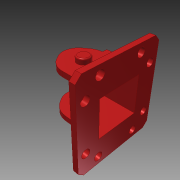
# Autodesk Inventor part: z_axis_cable_mount_b
Saved by Autodesk Inventor 2014 (Build 180170000, 170)
## iProperties
Created: 2013-12-04
Part Number: z_axis_cable_mount_b
Material: ABS Plastic
Document SubType Name: Modeling
Designer: buben
Density: 1.06 g/cm^3
Appearance: Light Red
Author: buben
Autodesk Inventor part; units mm, degrees
ref_plane "YZ Plane" through (0, 0, 0) normal (1, 0, 0) x (0, 1, 0)
sketch "Sketch1" plane through (0, 0, 0) normal (0, 0, 1) x (1, 0, 0)
  circle A0 centre (0, 0) radius 2.5
  circle A1 centre (20, 0) radius 2.5
  line L0 (7, 10) -> (20, 10)
  line L1 (7, -10) -> (20, -10)
  arc A2 (20, -10) -> (20, 10) centre (20, 0) ccw
  line L2 (7, 10) -> (7, 8)
  line L3 (7, -10) -> (7, -8)
  line L4 (7, 8) -> (0, 8)
  line L5 (7, -8) -> (0, -8)
  arc A3 (0, 8) -> (0, -8) centre (0, 0) ccw
  dimension "d0" = 5
  dimension "d1" = 20
  dimension "d2" = 10
  dimension "d3" = 2
  dimension "d4" = 13
  constraints: 12 end point, 4 centre point, 4 point on circle, 4 tangent, 3 parallel, 2 collinear, 2 concentric, 1 coincident, 1 equal radius, 1 horizontal, 1 horizontal alignment, 1 perpendicular
  measures "d0" diameter of A0
  measures "d1" distance of A1.centre point (0, 0)
  measures "d2" radius of A2
  measures "d3" distance of L0.start L2.end
  measures "d4" distance from line of L2 A1.centre
extrude "Extrusion1" add sketch "Sketch1" along normal blind 4
sketch "Sketch2" plane through (0, 0, 4) normal (0, 0, 1) x (1, 0, 0)
  circle A0 centre (0, 0) radius 2.5 projected
  line L0 (7, 8) -> (0, 8) projected
  arc A1 (0, 8) -> (0, -8) centre (0, 0) ccw projected
  line L1 (0, -8) -> (7, -8) projected
  line L2 (7, -10) -> (20, -10) projected
  line L3 (7, 8) -> (7, -8)
  line L4 (7, -8) -> (0, -8)
  line L5 (7, 8) -> (0, 8)
  arc A2 (0, 8) -> (0, -8) centre (0, 0) ccw
  constraints: 6 end point, 4 tangent, 2 collinear, 2 point on circle, 1 centre point, 1 perpendicular
extrude "Extrusion2" cut sketch "Sketch2" against normal blind 2
sketch "Sketch3" plane through (0, 0, 0) normal (0, 0, -1) x (-1, 0, 0)
  circle A0 centre (-20, 0) radius 2.5 projected
  circle A1 centre (0, 0) radius 2.5 projected
  line L0 (-7, 10) -> (-20, 10) projected
  arc A2 (-20, 10) -> (-20, -10) centre (-20, 0) ccw projected
  line L1 (-20, -10) -> (-7, -10) projected
  line L2 (-7, 8) -> (-7, 10) projected
  line L3 (-19, 10) -> (-19, 8)
  line L4 (-19, 8) -> (-11, 8)
  line L5 (-11, 8) -> (-11, -8)
  line L6 (-11, -8) -> (-19, -8)
  line L7 (-19, -8) -> (-19, -10)
  point P0 (-7, -8)
  dimension "d9" = 1
  dimension "d10" = 11
  constraints: 10 end point, 3 parallel, 2 horizontal alignment, 2 perpendicular, 2 point on line, 1 collinear
  measures "d9" distance from line of L3 A0.centre
  measures "d10" distance from line of A1.centre L5
extrude "Extrusion3" cut sketch "Sketch3" against normal blind 2 contours L3 L4 L5 L6 L7 L1 A2 L0
sketch "Sketch4" plane through (0, 0, 4) normal (0, 0, 1) x (1, 0, 0)
  line L0 (7, 10) -> (7, -10)
  circle A0 centre (0, 0) radius 2.5
  arc A1 (7, -8.485281) -> (7, 8.485281) centre (0, 0) ccw
  dimension "d15" = 11
  constraints: 2 point on circle, 2 point on line, 1 centre point, 1 coincident
  measures "d15" radius of A1
extrude "Extrusion4" cut sketch "Sketch4" against normal blind 2 contours A1 L0
sketch "Sketch5" plane through (0, 0, 0) normal (0, 0, -1) x (-1, 0, 0)
  line L0 (0, 8) -> (-7, 8) projected
  line L1 (-7, 10) -> (0, 10)
  line L2 (0, 10) -> (0, 8)
  line L3 (0, 8) -> (-7, 8)
  line L4 (-7, 8) -> (-7, 10)
  arc A0 (0, -8) -> (0, 8) centre (0, 0) ccw projected
  constraints: 8 end point, 2 parallel, 1 horizontal, 1 perpendicular, 1 point on line, 1 vertical alignment
extrude "Extrusion5" add sketch "Sketch5" against normal blind 2
sketch "Sketch6" plane through (0, 0, 0) normal (0, 0, -1) x (-1, 0, 0)
  line L0 (0, 10) -> (-19, 10) projected
  line L1 (-19, 8) -> (-20, 8)
  line L2 (-20, 8) -> (-20, 10)
  line L3 (-20, 10) -> (-19, 10)
  line L4 (-19, 10) -> (-19, 8)
  circle A0 centre (-20, 0) radius 2.5 projected
  constraints: 8 end point, 2 parallel, 1 collinear, 1 horizontal, 1 perpendicular, 1 vertical alignment
extrude "Extrusion6" add sketch "Sketch6" against normal blind 2 contours L1 L2 L3 L4
sketch "Sketch7" plane through (0, 0, 0) normal (0, 0, -1) x (-1, 0, 0)
  line L0 (-19, -8) -> (-19, -10)
  line L1 (-11, -8) -> (-19, -8)
  line L2 (-17.400642, -8) -> (-19, -9.162001)
  line L3 (-17.400642, -8) -> (-26.805206, 4.944272) construction
  line L4 (-26.805206, 4.944272) -> (-28.404564, 3.782271) construction
  line L5 (-28.404564, 3.782271) -> (-19, -9.162001) construction
  circle A0 centre (-20, 0) radius 2.5
  line L6 (-17.400642, -8) -> (-19, -8)
  line L7 (-19, -8) -> (-19, -9.162001)
  dimension "d21" = 16
  dimension "d22" = 8
  dimension "d23" = 36
  constraints: 12 end point, 3 perpendicular, 2 point on line, 1 collinear, 1 parallel
  measures "d21" distance of L2.start L3.end
  measures "d22" distance from line of A0.centre L4
  measures "d23" angle of L2 L1
extrude "Extrusion7" cut sketch "Sketch7" against normal blind 2 contours L1 L2 L0
sketch "Sketch9" plane through (0, 0, 2) normal (0, 0, 1) x (1, 0, 0)
  circle A0 centre (0, 0) radius 2.5
  arc A1 (11, 0) -> (7, 8.485281) centre (0, 0) ccw
  circle A2 centre (0, 0) radius 2.5
  constraints: 1 centre point, 1 coincident, 1 concentric
extrude "Extrusion8" add sketch "Sketch9" along normal mid plane 4
fillet "Fillet1" radius 0.5 1 edges at (-2.5, 0, 4)
sketch "Sketch10" plane through (0, 0, 0) normal (0, 0, -1) x (-1, 0, 0)
  arc A0 (0, -8) -> (0, 8) centre (0, 0) ccw
  line L0 (0, 10) -> (-20, 10)
  line L1 (4.702282, 6.472136) -> (11.174418, 1.769854)
  line L2 (11.174418, 1.769854) -> (6.472136, -4.702282)
  dimension "d30" = 144
  constraints: 4 end point, 2 point on circle, 2 tangent, 1 perpendicular
  measures "d30" angle of L1 L0
extrude "Extrusion9" add sketch "Sketch10" against normal blind 2
fillet "Fillet2" radius 6 1 edges at (-11.1744, 1.7699, 1)
ref_plane "Work Plane1" through (11, 0, 4) normal (1, 0, 0) x (0, 1, 0)
split "Split1" plane through (11, 0, 4) removes the side toward (1, 0, 0)
sketch "Sketch11" plane through (11, -10, 0) normal (1, 0, 0) x (0, 0, -1)
  line L0 (0, 20) -> (0, 0) projected
  line L1 (-4, 20) -> (0, 20) projected
  line L2 (-4, 10) -> (-4, 20) projected
  line L3 (-4, 0) -> (-4, 10) projected
  line L4 (0, 0) -> (-4, 0) projected
  point P0 (0, 10)
extrude "Extrusion10" add sketch "Sketch11" along normal blind 1
ref_plane "Work Plane2" through (0, 0, -7) normal (0, 0, -1) x (-1, 0, 0)
mirror "Mirror1" about plane through (0, 0, -7) normal (0, 0, -1)
sketch "Sketch12" plane through (0, 0, 0) normal (0, 0, -1) x (-1, 0, 0)
  line L0 (-12, -10) -> (-7, -10)
  line L1 (-7, -10) -> (-7, -8)
  arc A0 (4.702282, 6.472136) -> (0, 8) centre (0, 0) ccw
  line L2 (0, 8) -> (0, 10)
  line L3 (0, 10) -> (-12, 10)
  line L4 (-12, -10) -> (-12, 10)
  line L5 (0, 8) -> (-12, 8)
  line L6 (-7, -8) -> (-12, -8)
  constraints: 4 end point, 2 perpendicular, 2 point on line, 1 tangent
extrude "Extrusion11" add sketch "Sketch12" along normal blind 14
sketch "Sketch17" plane through (12, -10, 0) normal (1, 0, 0) x (0, 0, -1)
  line L0 (0, 2) -> (0, 18) projected
  line L1 (0, 18) -> (14, 18) projected
  line L2 (14, 2) -> (14, 18) projected
  line L3 (0, 2) -> (14, 2) projected
  line L4 (18, 20) -> (18, 0) projected
  line L5 (-4, 20) -> (18, 20) projected
  line L6 (-4, 20) -> (-4, 0) projected
  line L7 (-8, 26) -> (22, 26)
  line L8 (24, 24) -> (24, -4)
  line L9 (22, -6) -> (-8, -6)
  line L10 (-10, -4) -> (-10, 24)
  line L11 (-7, 23) -> (21, 23) construction
  line L12 (21, 23) -> (21, -3) construction
  line L13 (21, -3) -> (-7, -3) construction
  line L14 (-7, -3) -> (-7, 23) construction
  circle A0 centre (-2, -3) radius 1.6
  circle A1 centre (16, -3) radius 1.6
  circle A2 centre (21, 2) radius 1.6
  circle A3 centre (21, 18) radius 1.6
  circle A4 centre (16, 23) radius 1.6
  circle A5 centre (-2, 23) radius 1.6
  circle A6 centre (-7, 18) radius 1.6
  circle A7 centre (-7, 2) radius 1.6
  line L15 (-10, 24) -> (-8, 26)
  line L16 (-10, -4) -> (-8, -6)
  line L17 (22, -6) -> (24, -4)
  line L18 (24, 24) -> (22, 26)
  point P0 (0, 10)
  point P1 (-10, 26)
  point P2 (24, -6)
  point P3 (24, 26)
  point P4 (-10, -6)
  point P5 (-7, 10)
  point P6 (-4, 10)
  point P7 (7, 23)
  point P8 (7, 20)
  point P9 (24, 10)
  point P10 (21, 10)
  point P11 (7, -6)
  point P12 (7, -3)
  dimension "d73" = 3.2
  dimension "d74" = 5
  dimension "d75" = 5
  dimension "d76" = 5
  dimension "d77" = 5
  dimension "d78" = 5
  dimension "d79" = 5
  dimension "d80" = 5
  dimension "d81" = 5
  dimension "d82" = 3
  dimension "d83" = 3
  dimension "d84" = 2
  dimension "d85" = 2
  dimension "d86" = 2
  dimension "d87" = 2
  dimension "d88" = 2
  dimension "d89" = 2
  dimension "d90" = 2
  dimension "d91" = 2
  dimension "d92" = 3
  dimension "d93" = 3
  constraints: 24 end point, 16 point on line, 8 centre point, 8 midpoint, 7 equal radius, 4 parallel, 2 horizontal, 2 horizontal alignment, 2 perpendicular, 2 vertical alignment
  measures "d73" diameter of A0
  measures "d74" distance of L13.end A0.centre
  measures "d75" distance of L12.end A1.centre
  measures "d76" distance of L12.end A2.centre
  measures "d77" distance of L11.end A3.centre
  measures "d78" distance of A4.centre L11.end
  measures "d79" distance of L11.start A5.centre
  measures "d80" distance of L11.start A6.centre
  measures "d81" distance of L13.end A7.centre
  measures "d82" distance between parallel lines of L4 L12
  measures "d83" distance between parallel lines of L5 L11
  measures "d84" distance of L10.end point (-10, 26)
  measures "d85" distance of L7.start point (-10, 26)
  measures "d86" distance of L10.start point (-10, -6)
  measures "d87" distance of L9.end point (-10, -6)
  measures "d88" distance of L9.start point (24, -6)
  measures "d89" distance of L8.end point (24, -6)
  measures "d90" distance of L8.start point (24, 26)
  measures "d91" distance of L7.end point (24, 26)
  measures "d92" distance between parallel lines of L7 L11
  measures "d93" distance between parallel lines of L10 L14
extrude "Extrusion16" add sketch "Sketch17" along normal blind 2
equation "\"d75\" = d74"
equation "\"d76\" = d75"
equation "\"d77\" = d76"
equation "\"d78\" = d76"
equation "\"d79\" = d75"
equation "\"d80\" = d75"
equation "\"d81\" = d75"
equation "\"d85\" = d84"
equation "\"d86\" = d84"
equation "\"d87\" = d86"
equation "\"d88\" = d84"
equation "\"d89\" = d88"
equation "\"d90\" = d84"
equation "\"d91\" = d90"
body "Solid1"
